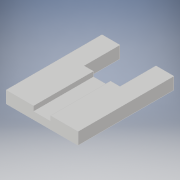
# Autodesk Inventor part: RS-RemovableFiber
Saved by Autodesk Inventor 2019 (Build 230136000, 136)
## iProperties
Created: 2019-06-18
Part Number: RS-RemovableFiber
Material: Generic
Document SubType Name: Modeling
Designer: aorfi
Density: 1 g/cm^3
Appearance: Default
Author: aorfi
Autodesk Inventor part; units mm, degrees
ref_plane "YZ Plane" through (0, 0, 0) normal (1, 0, 0) x (0, 1, 0)
ref_plane "XZ Plane" through (0, 0, 0) normal (0, 1, 0) x (-1, 0, 0)
ref_plane "XY Plane" through (0, 0, 0) normal (0, 0, 1) x (1, 0, 0)
sketch "Sketch1" plane through (0, 0, 0) normal (0, 1, 0) x (-1, 0, 0)
  line L0 (15, 20) -> (15, -20)
  line L1 (15, -20) -> (7.5, -20)
  line L2 (7.5, -20) -> (7.5, -5)
  line L3 (7.5, -5) -> (-7.5, -5)
  line L4 (-7.5, -5) -> (-7.5, -20)
  line L5 (-7.5, -20) -> (-15, -20)
  line L6 (-15, -20) -> (-15, 20)
  line L7 (-15, 20) -> (15, 20)
  point P0 (0, 0)
  point P1 (0, 20)
  point P2 (0, -5)
  point P3 (15, 0)
  dimension "d2" = 30
  dimension "d3" = 40
  dimension "d4" = 15
  dimension "d5" = 15
  constraints: 16 end point, 6 perpendicular, 3 midpoint, 2 point on line, 2 vertical alignment, 1 horizontal alignment, 1 vertical
  measures "d2" distance of L6.end L0.start
  measures "d3" distance of L0.start L0.end
  measures "d4" distance of L1.end L2.end
  measures "d5" distance of L2.end L3.end
extrude "Extrusion1" add sketch "Sketch1" along normal mid plane 3
sketch "Sketch2" plane through (0, 1.5, 0) normal (0, 1, 0) x (1, 0, 0)
  line L0 (3.5625, -20) -> (-3.5625, -20)
  line L1 (-3.5625, -20) -> (-3.5625, 5)
  line L2 (-3.5625, 5) -> (3.5625, 5)
  line L3 (3.5625, 5) -> (3.5625, -20)
  line L4 (3.5625, -20) -> (-3.5625, 5) construction
  line L5 (-3.5625, -20) -> (3.5625, 5) construction
  line L6 (-15, -20) -> (15, -20) projected
  line L7 (7.5, 5) -> (-7.5, 5) projected
  line L8 (-15, 20) -> (-15, -20) projected
  line L9 (-15, -20) -> (15, -20) projected
  line L10 (15, -20) -> (15, 20) projected
  line L11 (15, 20) -> (7.5, 20) projected
  line L12 (7.5, 20) -> (7.5, 5) projected
  line L13 (7.5, 5) -> (-7.5, 5) projected
  line L14 (-7.5, 5) -> (-7.5, 20) projected
  line L15 (-7.5, 20) -> (-15, 20) projected
  point P0 (0, 0)
  point P1 (0, -7.5)
  point P2 (0, -7.5)
  dimension "d8" = 7.125
  constraints: 12 end point, 3 midpoint, 2 collinear, 2 parallel, 1 horizontal, 1 perpendicular, 1 vertical alignment
  measures "d8" distance of L0.start L0.end
extrude "Extrusion2" add sketch "Sketch2" along normal blind 2 contours L3 L7 L12 L11 L10 L6 | L6 L8 L15 L14 L7 L1
body "Solid1"
